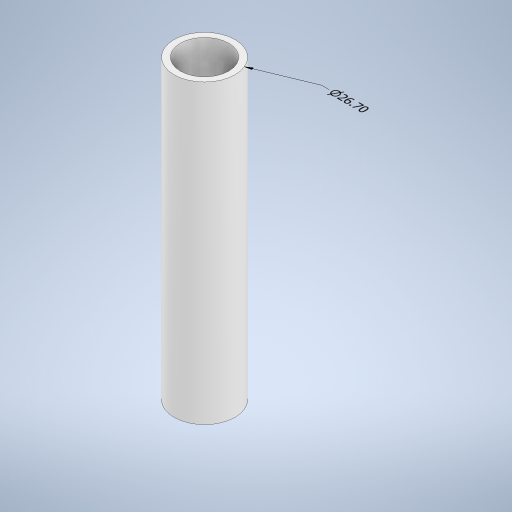
# Autodesk Inventor part: TuboMarcador
Saved by Autodesk Inventor 2023.1 (Build 271208000, 208)
## iProperties
Created: 2022-08-24
Part Number: TuboMarcador
Material: PVC-Piping
Document SubType Name: Modeling
Designer: Daniel Peña
Density: 1.4 g/cm^3
Appearance: Smooth - White
Author: Daniel Peña
Autodesk Inventor part; units mm, degrees
ref_plane "YZ Plane" through (0, 0, 0) normal (1, 0, 0) x (0, 1, 0)
ref_plane "XZ Plane" through (0, 0, 0) normal (0, 1, 0) x (-1, 0, 0)
ref_plane "XY Plane" through (0, 0, 0) normal (0, 0, 1) x (1, 0, 0)
sketch "Sketch1" plane through (0, 0, 0) normal (0, 0, 1) x (1, 0, 0)
  line L0 (13.35, -28.0978) -> (13.35, 101.9022)
  line L1 (0, 69.4184) -> (0, -28.0978)
  line L2 (10.6, -28.0978) -> (10.6, 101.9022)
  line L3 (10.6, -28.0978) -> (13.35, -28.0978)
  line L4 (10.6, 101.9022) -> (13.35, 101.9022)
  point P0 (0, 0)
  dimension "d9" = 21.2
  dimension "d10" = 26.7
  dimension "d11" = 130
  constraints: 10 end point, 2 horizontal, 2 parallel
  measures "d9" diameter of L2 L1
  measures "d10" diameter of L0 L1
  measures "d11" distance of L0.start L0.end
revolve "Revolution1" add sketch "Sketch1" angle 360 about axis through (0, 69.4184, 0) along (0, -1, 0)
body "Solid1"
